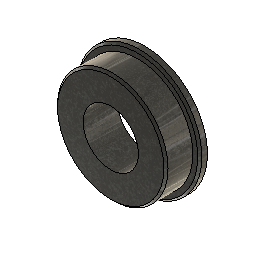
ROLAMENTO v1 (Autodesk Fusion 360 design; units mm, degrees)
Autodesk Fusion 360 part; units mm, degrees
sketch "Esboço1" plane through (0, 0, 0) normal (0, 1, 0) x (1, 0, 0)
  circle A0 centre (0, 0) radius 8
  circle A1 centre (0, 0) radius 4
  dimension "d1" = 16
  dimension "d2" = 8
  constraint coincident A0.centre A1.centre
  measures "d1" diameter of A0
  measures "d2" diameter of A1
extrude "Extrusão1" add sketch "Esboço1" along normal blind 3.9
sketch "Esboço2" plane through (0, 3.9, 0) normal (0, 1, 0) x (-1, 0, 0)
  circle A0 centre (0, 0) radius 4
  circle A1 centre (0, 0) radius 8
  circle A2 centre (0, 0) radius 9
  dimension "d5" = 18
  constraint concentric A0 A2
  measures "d5" diameter of A2
extrude "Extrusão2" add sketch "Esboço2" along normal blind 1.1 contours A1 | A2
chamfer "Chanfro1" distance 0.3 angle 45 1 edges at (-7.4586, 0, 2.8929)
chamfer "Chanfro2" distance 0.3 angle 45 1 edges at (8.3909, 3.9, -3.2545)
